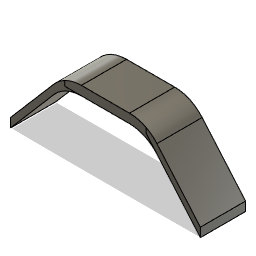
Landing Gear Conventional v1 (Autodesk Fusion 360 design; units mm, degrees)
Autodesk Fusion 360 part; units mm, degrees
sketch "Sketch1" plane through (0, 0, 0) normal (1, 0, 0) x (0, 0, -1)
  line L0 (-25, 5) -> (0, 5)
  line L1 (0, 5) -> (0, 0)
  line L2 (0, 0) -> (-25, 0)
  line L3 (-25, 0) -> (-25, 5)
  line L4 (-25, 40, 30) -> (0, 40, 30)
  line L5 (0, 40, 30) -> (0, 35, 30)
  line L6 (0, 35, 30) -> (-25, 35, 30)
  line L7 (-25, 35, 30) -> (-25, 40, 30)
  constraint horizontal L0
  constraint vertical L1
  constraint horizontal L2
  constraint vertical L3
  constraint coincident L1.end L2.start
loft "Loft1" add profiles "Sketch1", "Sketch1" section 1 section 2 contours L4 L5 L6 L7 in plane through (30, 0, 0) normal (1, 0, 0)
sketch "Sketch2" plane through (0, 0, 0) normal (1, 0, 0) x (0, 0, -1)
  line L0 (-25, 40, 75) -> (0, 40, 75)
  line L1 (0, 40, 75) -> (0, 35, 75)
  line L2 (0, 35, 75) -> (-25, 35, 75)
  line L3 (-25, 35, 75) -> (-25, 40, 75)
loft "Loft2" add profiles "Sketch2" section 1 contours L0 L1 L2 L3 in plane through (75, 0, 0) normal (1, 0, 0) section 2 face at (30, 36.6667, 16.6667)
sketch "Sketch3" plane through (75, 0, 0) normal (1, 0, 0) x (0, 0, -1)
  line L0 (-25, 35) -> (0, 35)
  line L1 (0, 35) -> (0, 40)
  line L2 (0, 40) -> (-25, 40)
  line L3 (-25, 40) -> (-25, 35)
  line L4 (-25, 5, 30) -> (0, 5, 30)
  line L5 (0, 5, 30) -> (0, 0, 30)
  line L6 (0, 0, 30) -> (-25, 0, 30)
  line L7 (-25, 0, 30) -> (-25, 5, 30)
loft "Loft3" add profiles "Sketch3", "Sketch3" section 1 contours L4 L5 L6 L7 in plane through (105, 0, 0) normal (1, 0, 0) section 2
fillet "Fillet1" radius 20 4 edges at (75, 40, 12.5) (30, 40, 12.5) (30, 35, 12.5) (75, 35, 12.5)
